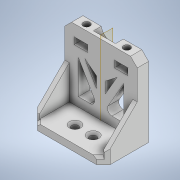
# Autodesk Inventor part: halter1
Saved by Autodesk Inventor 2022 (Build 260153000, 153)
## iProperties
Created: 2022-11-24
Part Number: halter1
Material: Generisch
Document SubType Name: Modeling
Designer: Friedrich Walmrath
Density: 1 g/cm^3
Appearance: Vorgabe
Author: Friedrich Walmrath
Autodesk Inventor part; units mm, degrees
ref_plane "YZ Plane" through (0, 0, 0) normal (1, 0, 0) x (0, 1, 0)
ref_plane "XZ Plane" through (0, 0, 0) normal (0, 1, 0) x (-1, 0, 0)
ref_plane "XY Plane" through (0, 0, 0) normal (0, 0, 1) x (1, 0, 0)
sketch "Skizze1" plane through (0, 0, 0) normal (0, 0, 1) x (1, 0, 0)
  circle A0 centre (0, 0) radius 5
  line L0 (4.899, -1) -> (16.009, -1)
  line L1 (16.009, -1) -> (16.009, -35)
  line L2 (16.009, -35) -> (0, -35)
  line L3 (0, -35) -> (0, -1)
  line L4 (0, -1) -> (4.899, -1)
  point P0 (0, -5)
  dimension "d0" = 10
  dimension "d1" = 11.11
  dimension "d2" = 1
  dimension "d3" = 35
  constraints: 10 end point, 3 perpendicular, 1 coincident, 1 horizontal, 1 point on line, 1 vertical alignment, 3 other
  measures "d1" distance of L0.start L0.end
  measures "d2" distance of L3.end point (0, 0)
  measures "d3" distance from line of L2 point (0, 0)
extrude "Extrusion1" add sketch "Skizze1" along normal blind 5 contours L0 L1 L2 L3 A0
mirror "Spiegeln1" about plane through (0, -5, 0) normal (-1, 0, 0) of "Extrusion1"
sketch "Skizze2" plane through (-16.009, -1, 0) normal (0, 1, 0) x (1, 0, 0)
  circle A0 centre (7.11, -2.5) radius 1.5
  line L0 (0, 0) -> (11.11, 0) projected
  line L1 (11.11, 0) -> (11.11, -5) projected
  point P0 (16.009, 0)
  dimension "d7" = 3
  dimension "d8" = 2.5
  dimension "d9" = 4
  constraints: 1 centre point
  measures "d7" diameter of A0
  measures "d8" distance from line of L0 A0.centre
  measures "d9" distance from line of A0.centre L1
extrude "Extrusion2" cut sketch "Skizze2" against normal blind 5
sketch "Skizze3" plane through (0, 0, 5) normal (0, 0, 1) x (1, 0, 0)
  line L0 (-11.899, -6) -> (-5.899, -6)
  line L1 (-5.899, -6) -> (-5.899, -9)
  line L2 (-5.899, -9) -> (-11.899, -9)
  line L3 (-11.899, -9) -> (-11.899, -6)
  line L4 (-16.009, -1) -> (-4.899, -1) projected
  line L5 (-10.399, -6) -> (-7.399, -6) projected
  point P0 (0, 0)
  point P1 (-8.899, -6)
  point P2 (-8.899, -6)
  point P3 (-8.899, -9)
  point P4 (-8.899, -6)
  dimension "d12" = 6
  dimension "d13" = 3
  dimension "d14" = 5
  dimension "d15" = 4
  constraints: 8 end point, 3 midpoint, 2 parallel, 1 coincident, 1 horizontal, 1 perpendicular, 1 vertical alignment
  measures "d12" distance of L1.end L2.end
  measures "d13" distance of L0.end L1.end
  measures "d14" distance between parallel lines of L0 L4
  measures "d15" horizontal distance of L4.end point (-8.899, -6)
extrude "Extrusion3" cut sketch "Skizze3" along normal through all both and the other way through all
ref_plane "Arbeitsebene1" through (0, -35, 0) normal (1, 0, 0) x (0, 0, -1)
mirror "Spiegeln2" about plane through (0, -35, 0) normal (1, 0, 0) of "Extrusion3", "Extrusion2"
sketch "Skizze4" plane through (0, 0, 5) normal (0, 0, 1) x (1, 0, 0)
  arc A0 (-4.899, -1) -> (4.899, -1) centre (0, 0) ccw projected
  line L0 (-16.009, -1) -> (-4.899, -1) projected
  line L1 (-4.899, -1) -> (4.899, -1)
  constraints: 2 end point, 1 collinear
extrude "Extrusion4" add sketch "Skizze4" against normal blind 1.5
sketch "Skizze5" plane through (16.009, -35, 0) normal (1, 0, 0) x (0, 0, -1)
  line L0 (-5, 0) -> (-5, 34) projected
  line L1 (0, 0) -> (-5, 0) projected
  line L2 (-5, 0) -> (-20, 0)
  line L3 (-20, 0) -> (-20, 3)
  line L4 (-20, 3) -> (-5, 3)
  line L5 (-5, 3) -> (-5, 0)
  point P0 (0, 35)
  point P1 (-5, 3)
  dimension "d20" = 15
  dimension "d21" = 3
  constraints: 8 end point, 2 parallel, 1 horizontal, 1 perpendicular
  measures "d20" distance of L3.end L4.end
  measures "d21" distance of L2.end L3.end
extrude "Extrusion5" add sketch "Skizze5" against normal up to surface (32.018 mm away)
sketch "Skizze6" plane through (-16.009, -35, 0) normal (-1, 0, 0) x (0, 0, 1)
  line L0 (20, 3) -> (20, 0) projected
  line L1 (20, 3) -> (5, 18)
  line L2 (5, 3) -> (5, 34) projected
  line L3 (20, 3) -> (5, 3)
  point P0 (0, 35)
  dimension "d24" = 15
  constraints: 4 end point, 1 perpendicular, 1 point on line
  measures "d24" distance of L2.start L1.end
extrude "Extrusion6" add sketch "Skizze6" against normal blind 2
mirror "Spiegeln3" about plane through (0, -35, 0) normal (1, 0, 0) of "Extrusion6"
sketch "Skizze7" plane through (-14.009, -32, 20) normal (0, 1, 0) x (1, 0, 0)
  circle A0 centre (10, 7.5) radius 1.5
  circle A1 centre (18.018, 7.5) radius 1.5
  line L0 (28.018, 0) -> (0, 0) projected
  line L1 (0, 15) -> (0, 0) projected
  line L2 (28.018, 15) -> (28.018, 0) projected
  point P0 (14.009, 20)
  dimension "d27" = 3
  dimension "d28" = 3
  dimension "d29" = 7.5
  dimension "d30" = 10
  dimension "d31" = 10
  constraints: 2 centre point, 1 horizontal alignment
  measures "d27" diameter of A0
  measures "d28" diameter of A1
  measures "d29" distance from line of L0 A0.centre
  measures "d30" distance from line of A0.centre L1
  measures "d31" distance from line of L2 A1.centre
extrude "Extrusion7" cut sketch "Skizze7" along normal through all both and the other way through all
chamfer "Fase1" distance 1 angle 45 2 edges at (-5.509, -32, 12.5) (2.509, -32, 12.5)
sketch "Skizze10" plane through (0, 0, 5) normal (0, 0, 1) x (1, 0, 0)
  line L0 (14.009, -17) -> (16.009, -17) projected
  line L1 (16.009, -17) -> (16.009, -1) projected
  line L2 (16.009, -1) -> (-16.009, -1) projected
  line L3 (-16.009, -17) -> (-16.009, -1) projected
  line L4 (-16.009, -17) -> (-14.009, -17) projected
  line L5 (-14.009, -17) -> (-14.009, -32) projected
  line L6 (-14.009, -32) -> (14.009, -32) projected
  line L7 (14.009, -32) -> (14.009, -17) projected
  line L8 (5.899, -6) -> (11.899, -6) projected
  line L9 (11.899, -6) -> (11.899, -9) projected
  line L10 (11.899, -9) -> (5.899, -9) projected
  line L11 (5.899, -9) -> (5.899, -6) projected
  line L12 (-11.899, -9) -> (-11.899, -6) projected
  line L13 (-11.899, -6) -> (-5.899, -6) projected
  line L14 (-5.899, -6) -> (-5.899, -9) projected
  line L15 (-5.899, -9) -> (-11.899, -9) projected
  line L16 (-12.009, -5) -> (12.009, -5)
  line L17 (12.009, -5) -> (12.009, -13)
  line L18 (12.009, -13) -> (10.009, -13)
  line L19 (10.009, -13) -> (10.009, -28)
  line L20 (10.009, -28) -> (-10.009, -28)
  line L21 (-10.009, -28) -> (-10.009, -13)
  line L22 (-10.009, -13) -> (-12.009, -13)
  line L23 (-12.009, -13) -> (-12.009, -5)
  line L24 (-10.009, -13) -> (-1.3487, -28)
  line L25 (-7.1222, -12) -> (-2, -20.872)
  line L26 (-2, -20.872) -> (-2, -16)
  line L27 (-2, -16) -> (-7.1222, -12)
  line L28 (0, 7) -> (0, -42) projected
  point P0 (0, 0)
  dimension "d37" = 4
  dimension "d38" = 30
  dimension "d39" = 2
  dimension "d40" = 3
  dimension "d41" = 3
  dimension "d42" = 7
  constraints: 24 end point, 1 parallel, 1 point on line, 1 vertical, 7 other
  measures "d37" distance between parallel lines of L2 L16
  measures "d38" angle of L21 L24
  measures "d39" distance between parallel lines of L26 L28
  measures "d40" distance between parallel lines of L24 L25
  measures "d41" distance from line of L25.start L15
  measures "d42" vertical distance of L26.end L14.end
extrude "Extrusion8" cut sketch "Skizze10" along normal through all both and the other way through all contours L20 L21 L24 | L27 L26 L25
mirror "Spiegeln4" about plane through (0, -35, 0) normal (1, 0, 0) of "Extrusion8"
chamfer "Fase2" distance 3 angle 45 4 edges at (16.009, -1, 2.5) (-16.009, -1, 2.5) (-16.009, -33.5, 20) (16.009, -33.5, 20)
chamfer "Fase3" distance 1 angle 45 4 edges at (-14.009, -31.5, 19) (-13.509, -32, 19.5) (13.509, -32, 19.5) (14.009, -31.5, 19)
fillet "Rundung1" radius 2 2 edges at (-1.3487, -28, 2.5) (1.3487, -28, 2.5)
